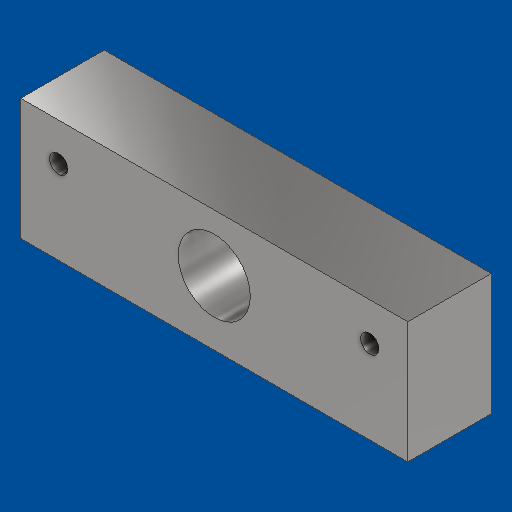
# Autodesk Inventor part: Micrometer_Holder
Saved by Autodesk Inventor 2025.1 (Build 291241000, 241)
## iProperties
Created: 2024-12-27
Part Number: Micrometer_Holder
Material: Steel, Carbon
Document SubType Name: Modeling
Designer: konch
Density: 7.85 g/cm^3
Appearance: Semi-Polished
Mass: 8.05404 g
Surface Area: 34.6545 cm^2
Volume: 8.05404 cm^3
Author: konch
Autodesk Inventor part; units mm, degrees
ref_plane "YZ Plane" through (0, 0, 0) normal (1, 0, 0) x (0, 1, 0)
ref_plane "XZ Plane" through (0, 0, 0) normal (0, 1, 0) x (-1, 0, 0)
ref_plane "XY Plane" through (0, 0, 0) normal (0, 0, 1) x (1, 0, 0)
sketch "Sketch1" plane through (0, 0, 0) normal (0, 0, 1) x (1, 0, 0)
  line L0 (0, 0) -> (51, 0)
  line L1 (0, 0) -> (0, 16)
  line L2 (0, 16) -> (51, 16)
  line L3 (51, 16) -> (51, 0)
  line L4 (0, 0) -> (0, 8.5) construction
  line L5 (0, 8.5) -> (51, 8.5) construction
  line L6 (25.5, 16) -> (25.5, 0) construction
  circle A0 centre (25.5, 8.5) radius 4.75
  dimension "d1" = 16
  dimension "d2" = 51
  dimension "d5" = 8.5
  dimension "d6" = 9.5
  constraints: 14 end point, 3 midpoint, 3 point on line, 2 horizontal, 1 centre point, 1 perpendicular, 1 vertical
  measures "d1" distance of L0.start L1.end
  measures "d2" distance of L1.end L2.end
  measures "d5" distance of L0.start L4.end
  measures "d6" diameter of A0
extrude "Extrusion1" add sketch "Sketch1" along normal blind 11
sketch "Sketch3" plane through (0, 0, 0) normal (0, 0, -1) x (-1, 0, 0)
  circle A0 centre (-46, 11) radius 1.2 projected
  circle A1 centre (-5, 11) radius 2.2 projected
  point P0 (0, 0)
  constraints: 2 coincident
hole "Hole2" at (46, 11, 0) at (5, 11, 0) direction (0, 0, 1) diameter 2.4 end through all counterbore diameter 4.4 counterbore depth 2
body "Solid1"
